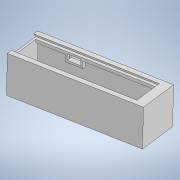
# Autodesk Inventor part: battery and buck converter enclosure
Saved by Autodesk Inventor 2022 (Build 260153000, 153)
## iProperties
Created: 2021-10-07
Part Number: battery and buck converter enclosure
Material: Generic
Document SubType Name: Modeling
Designer: tecware
Density: 1 g/cm^3
Appearance: Default
Author: tecware
## iProperties of the stored document battery and buck converter enclosure_3DPrint.ipt
Created: 2021-10-07
Part Number: battery and buck converter enclosure_3DPrint
Material: Generic
Document SubType Name: Modeling
Designer: tecware
Density: 1 g/cm^3
Appearance: Default
Author: tecware
Autodesk Inventor part; units mm, degrees
ref_plane "YZ Plane" through (0, 0, 0) normal (1, 0, 0) x (0, 1, 0)
ref_plane "XZ Plane" through (0, 0, 0) normal (0, 1, 0) x (-1, 0, 0)
sketch "Sketch1" plane through (0, 0, 0) normal (0, 1, 0) x (-1, 0, 0)
  line L0 (90, -19.5) -> (-30, -19.5)
  line L1 (-30, -19.5) -> (-30, 15.5)
  line L2 (-30, 15.5) -> (90, 15.5)
  line L3 (90, 15.5) -> (90, -19.5)
  dimension "d0" = 120
  dimension "d1" = 35
  constraints: 8 end point, 2 parallel, 1 horizontal, 1 perpendicular
  measures "d0" distance of L1.end L2.end
  measures "d1" distance of L0.end L1.end
extrude "Main Body" add sketch "Sketch1" along normal blind 35
shell "Main Shell" thickness 2 outward yes removed faces 1 at (-50, 35, 3.8333)
ref_plane "Work Plane2" through (-92, -2, -2) normal (0, 0, 1) x (1, 0, 0)
sketch "Sketch19" plane through (-90, 0, -19.5) normal (1, 0, 0) x (0, 0, -1)
  line L0 (-35, 35) -> (-35, 31)
  line L1 (-35, 35) -> (-32, 35)
  line L2 (2, 35) -> (-37, 35) projected
  line L3 (-35, 31) -> (-32, 35)
  line L4 (-17.5, 35) -> (-17.5, 25)
  line L5 (-35, 31) -> (-32, 31)
  line L6 (-32, 31) -> (-32, 28)
  line L7 (-32, 28) -> (-35, 28)
  line L8 (-35, 28) -> (-35, 31)
  line L9 (0, 0) -> (-35, 0) projected
  line L10 (0, 0) -> (0, 35) projected
  line L11 (-35, 35) -> (0, 35) projected
  line L12 (-35, 0) -> (-35, 35) projected
  line L13 (0, 35) -> (0, 31)
  line L14 (0, 35) -> (-3, 35)
  line L15 (0, 31) -> (-3, 35)
  line L16 (0, 31) -> (-3, 31)
  line L17 (-3, 31) -> (-3, 28)
  line L18 (-3, 28) -> (0, 28)
  line L19 (0, 28) -> (0, 31)
  line L20 (-35, 35) -> (0, 35) projected
  point P0 (-19.5, 0)
  point P1 (-35, 33)
  point P2 (0, 33)
  point P3 (-3, 35)
  dimension "d107" = 3
  dimension "d108" = 4
  dimension "d109" = 3
  dimension "d110" = 3
  constraints: 30 end point, 8 symmetric about line, 3 point on line, 2 horizontal, 2 midpoint, 2 parallel, 2 vertical, 1 perpendicular
  measures "d107" distance of L0.start L1.end
  measures "d108" distance of L0.start L0.end
  measures "d109" distance of L7.end L0.end
  measures "d110" distance of L6.end L7.end
extrude "Rail" add sketch "Sketch19" along normal up to surface (122 mm away) contours L1 L3 L0 | L5 L6 L7 L8 | L2 L10 L15 | L10 L18 L17 L16
sketch "Sketch27" plane through (-92, -2, -2) normal (0, 0, 1) x (1, 0, 0)
  line L0 (124, 0) -> (124, 37) projected
  line L1 (122, 33) -> (2, 33) projected
  line L2 (2, 37) -> (122, 37) projected
  line L3 (122, 37) -> (122.5, 37)
  line L4 (124, 37) -> (0, 37) projected
  line L5 (122.5, 37) -> (114.5, 37)
  line L6 (118.5, 37) -> (118.5, 35)
  line L7 (118.0528, 35.2236) -> (114.5, 37)
  line L8 (118.9472, 35.2236) -> (122.5, 37)
  arc A0 (118.0528, 35.2236) -> (118.9472, 35.2236) centre (118.5, 36.118) ccw
  point P0 (92, 2)
  dimension "d157" = 0.5
  dimension "d158" = 8
  dimension "d159" = 2
  dimension "d160" = 1
  constraints: 10 end point, 4 point on line, 2 point on circle, 2 tangent, 1 centre point, 1 midpoint, 1 vertical
  measures "d157" distance of L2.end L3.end
  measures "d158" distance of L3.end L5.end
  measures "d159" distance of L6.start L6.end
  measures "d160" radius of A0
extrude "Groove for snap fit" add sketch "Sketch27" along normal mid plane 39
fillet "Fillet3" radius 0.75 1 edges at (30, 34.75, -2)
sketch "Sketch3" plane through (-90, 0, -19.5) normal (0, 0, 1) x (1, 0, 0)
  line L0 (28.9, 29) -> (41.1, 29)
  line L1 (41.1, 29) -> (41.1, 23.5)
  line L2 (41.1, 23.5) -> (28.9, 23.5)
  line L3 (28.9, 23.5) -> (28.9, 29)
  line L4 (0, 35) -> (120, 35) projected
  point P0 (90, 0)
  dimension "d9" = 12.2
  dimension "d10" = 5.5
  dimension "d75" = 6
  constraints: 8 end point, 2 parallel, 1 horizontal, 1 perpendicular
  measures "d9" distance of L1.end L2.end
  measures "d10" distance of L0.end L1.end
  measures "d75" distance between parallel lines of L4 L0
extrude "Switch Cutout" cut sketch "Sketch3" along normal mid plane 16
sketch "Sketch8" plane through (-90, 0, -19.5) normal (0, 0, 1) x (1, 0, 0)
  line L0 (28.9, 23.5) -> (41.1, 23.5) projected
  line L1 (29, 35.5) -> (41.1, 35.5)
  line L2 (41.1, 35.5) -> (41.1, 23.5)
  line L3 (41.1, 23.5) -> (29, 23.5)
  line L4 (29, 23.5) -> (29, 35.5)
  line L5 (27, 35.5) -> (43.1, 35.5)
  line L6 (43.1, 35.5) -> (43.1, 21.5)
  line L7 (43.1, 21.5) -> (27, 21.5)
  line L8 (27, 21.5) -> (27, 35.5)
  line L9 (27, 29) -> (43.1, 29)
  point P0 (90, 0)
  point P1 (29, 23.5)
  point P2 (41.1, 29)
  point P3 (29, 29)
  dimension "d40" = 2
  dimension "d41" = 2
  dimension "d42" = 2
  dimension "d77" = 5.5
  constraints: 18 end point, 4 parallel, 3 perpendicular, 2 horizontal, 2 point on line
  measures "d40" distance between parallel lines of L4 L8
  measures "d41" distance between parallel lines of L6 L2
  measures "d42" distance between parallel lines of L0 L7
  measures "d77" distance between parallel lines of L9 L0
extrude "Switch Holder" add sketch "Sketch8" along normal blind 3 contours L0 L2 L9 L6 L7 L8 L4
sketch "Sketch23" plane through (-90, 0, 15.5) normal (1, 0, 0) x (0, 0, -1)
  line L0 (3, 28) -> (0, 28) projected
  line L1 (0, 0) -> (0, 28) projected
  line L2 (35, 0) -> (0, 0) projected
  line L3 (35, 0) -> (35, 28) projected
  line L4 (35, 28) -> (32, 28) projected
  line L5 (32, 28) -> (32, 31) projected
  line L6 (32, 31) -> (35, 31) projected
  line L7 (35, 31) -> (32, 35) projected
  line L8 (3, 35) -> (32, 35) projected
  line L9 (3, 35) -> (0, 31) projected
  line L10 (0, 31) -> (3, 31) projected
  line L11 (3, 31) -> (3, 28) projected
  line L12 (3, 31) -> (3, 28) projected
  line L13 (3, 31) -> (32, 31)
  line L14 (32, 28) -> (32, 31) projected
  line L15 (32, 30) -> (3, 30)
  point P0 (15.5, 0)
  point P1 (3, 30)
  dimension "d185" = 1
  constraints: 4 end point, 2 perpendicular, 2 point on line
  measures "d185" distance between parallel lines of L13 L15
extrude "Cutout for cover" cut sketch "Sketch23" against normal up to next contours L10 L9 L8 L7 L6 L13
equation "\"d41\" = d40"
equation "\"d42\" = d40"
equation "\"d77\" = d10"
equation "\"d28\" = 55deg"
equation "\"Sketch5_Pitch\" = 3"
equation "\"d60\" = 55deg"
equation "\"Sketch10_Pitch\" = 3"
equation "\"d91\" = 55deg"
equation "\"Sketch14_Pitch\" = 3"
equation "\"d123\" = 55deg"
equation "\"Sketch20_Pitch\" = 3"
equation "\"d173\" = 55deg"
equation "\"Sketch29_Pitch\" = 3"
equation "\"d193\" = 55deg"
equation "\"Sketch32_Pitch\" = 3"
body "Solid1"
